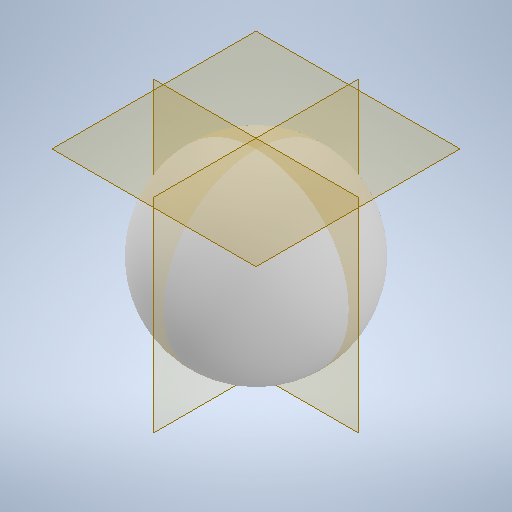
# Autodesk Inventor part: caster_wheel_link
Saved by Autodesk Inventor 2025.2 (Build 292293000, 293)
## iProperties
Created: 2025-11-14
Part Number: caster_wheel_link
Material: Genérico
Document SubType Name: Modeling
Designer: igles
Density: 1 g/cm^3
Appearance: Valor por defecto
Author: igles
Autodesk Inventor part; units mm, degrees
sketch "Boceto1" plane through (0, 0, 0) normal (1, 0, 0) x (0, 1, 0)
  line L0 (0, 0) -> (-96.5, 0)
  arc A0 (0, 0) -> (-96.5, 0) centre (-48.25, 0) ccw
  line L1 (-48.25, 0) -> (-96.5, 0) construction
  line L2 (-48.25, 0) -> (0, 0) construction
  dimension "d1" = 180
  constraints: 6 end point, 2 point on circle, 1 centre point, 1 horizontal
  measures "d1" angle of L1 L2
revolve "Revolución1" add sketch "Boceto1" angle 360 about axis through (0, 0, 0) along (0, -1, 0)
